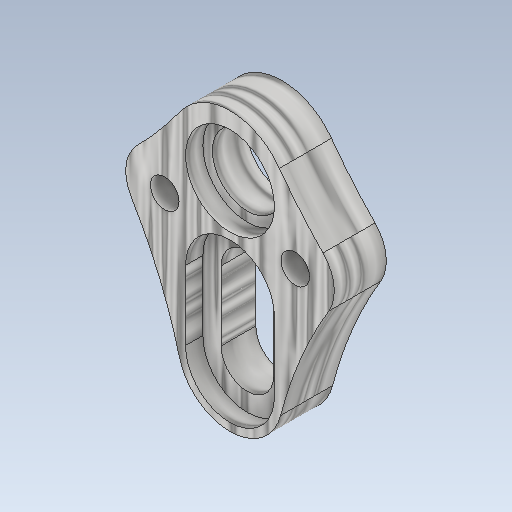
# Autodesk Inventor part: 横回転スライダー
Saved by Autodesk Inventor 2020 (Build 240168000, 168)
## iProperties
Created: 2019-09-03
Part Number: 横回転スライダー
Material: アルミニウム 7075
Document SubType Name: Modeling
Designer: tanjihayato
Density: 2.81 g/cm^3
Appearance: サテン - ブラシ仕上げ 重厚
Mass: 5.38037 g
Surface Area: 17.5615 cm^2
Volume: 1.91472 cm^3
Author: tanjihayato
Autodesk Inventor part; units mm, degrees
ref_plane "YZ Plane" through (0, 0, 0) normal (1, 0, 0) x (0, 1, 0)
ref_plane "XZ Plane" through (0, 0, 0) normal (0, 1, 0) x (-1, 0, 0)
ref_plane "XY Plane" through (0, 0, 0) normal (0, 0, 1) x (1, 0, 0)
sketch "スケッチ1" plane through (0, 0, 0) normal (0, 0, 1) x (1, 0, 0)
  circle A0 centre (0, 0) radius 4.025
  arc A1 (5.7008, 4.1051) -> (-5.7008, 4.1051) centre (0, 0) ccw
  line L0 (0, -11) -> (0, -19) construction
  line L1 (-3.025, -11) -> (-3.025, -19)
  line L2 (3.025, -19) -> (3.025, -11)
  arc A2 (3.025, -11) -> (-3.025, -11) centre (0, -11) ccw
  arc A3 (-3.025, -19) -> (3.025, -19) centre (0, -19) ccw
  arc A4 (-5.831, -20.5165) -> (5.831, -20.5165) centre (0, -19) ccw
  circle A5 centre (-7.525, -5) radius 1.65
  circle A6 centre (7.525, -5) radius 1.65
  line L3 (-7.525, -5) -> (7.525, -5) construction
  arc A7 (-10.7246, -1.8358) -> (-11.3806, -7.3203) centre (-7.525, -5) ccw
  arc A8 (-10.7246, -1.8358) -> (-5.7008, 4.1051) centre (-46.2759, 33.3226) ccw
  arc A9 (5.7008, 4.1051) -> (10.7246, -1.8358) centre (46.2759, 33.3226) ccw
  arc A10 (-5.831, -20.5165) -> (-11.3806, -7.3203) centre (-54.2212, -33.1019) ccw
  arc A11 (11.3806, -7.3203) -> (5.831, -20.5165) centre (54.2212, -33.1019) ccw
  arc A12 (11.3806, -7.3203) -> (10.7246, -1.8358) centre (7.525, -5) ccw
  point P0 (0, -15)
  dimension "d0" = 8.05
  dimension "d1" = 3
  dimension "d2" = 8
  dimension "d3" = 6.05
  dimension "d4" = 19
  dimension "d6" = 3.3
  dimension "d7" = 3.3
  dimension "d8" = 9
  dimension "d10" = 100
  dimension "d11" = 100
  dimension "d12" = 50
  dimension "d13" = 50
  dimension "d14" = 4.5
  dimension "d15" = 3
  dimension "d22" = 5
  constraints: 20 point on circle, 14 tangent, 13 centre point, 10 end point, 3 coincident, 1 horizontal, 1 midpoint, 1 parallel, 1 point on line, 1 vertical
  measures "d0" diameter of A0
  measures "d1" radial gap between concentric circles of A0 A1
  measures "d2" distance of L0.start L0.end
  measures "d3" diameter of A3
  measures "d4" distance of L0.end point (0, 0)
  measures "d6" diameter of A5
  measures "d7" diameter of A6
  measures "d8" diameter of A7
  measures "d10" diameter of A9
  measures "d11" diameter of A8
  measures "d12" radius of A11
  measures "d13" radius of A10
  measures "d14" radius of A12
  measures "d15" radial gap between concentric circles of A4 A3
  measures "d22" distance from line of L3 point (0, 0)
extrude "押し出し1" add sketch "スケッチ1" along normal blind 6
sketch "スケッチ2" plane through (0, 0, 6) normal (0, 0, 1) x (1, 0, 0)
  arc A0 (3.025, -11) -> (-3.025, -11) centre (0, -11) ccw projected
  line L0 (3.025, -11) -> (3.025, -19) projected
  arc A1 (-3.025, -19) -> (3.025, -19) centre (0, -19) ccw projected
  line L1 (-3.025, -19) -> (-3.025, -11) projected
  circle A2 centre (0, 0) radius 4.025 projected
  circle A3 centre (7.525, -5) radius 1.65 projected
  circle A4 centre (-7.525, -5) radius 1.65 projected
  arc A5 (-5.831, -20.5165) -> (5.831, -20.5165) centre (0, -19) ccw projected
  arc A6 (11.3806, -7.3203) -> (5.831, -20.5165) centre (54.2212, -33.1019) ccw projected
  arc A7 (11.3806, -7.3203) -> (10.7246, -1.8358) centre (7.525, -5) ccw projected
  arc A8 (5.7008, 4.1051) -> (10.7246, -1.8358) centre (46.2759, 33.3226) ccw projected
  arc A9 (5.7008, 4.1051) -> (-5.7008, 4.1051) centre (0, 0) ccw projected
  arc A10 (-10.7246, -1.8358) -> (-5.7008, 4.1051) centre (-46.2759, 33.3226) ccw projected
  arc A11 (-10.7246, -1.8358) -> (-11.3806, -7.3203) centre (-7.525, -5) ccw projected
  arc A12 (-5.831, -20.5165) -> (-11.3806, -7.3203) centre (-54.2212, -33.1019) ccw projected
  circle A13 centre (0, 0) radius 5.125
  arc A14 (5.125, -11) -> (-5.125, -11) centre (0, -11) ccw
  line L2 (5.125, -11) -> (5.125, -19)
  arc A15 (-5.125, -19) -> (5.125, -19) centre (0, -19) ccw
  line L3 (-5.125, -19) -> (-5.125, -11)
  dimension "d18" = 1.1
  dimension "d23" = 5.125
  constraints: 4 end point, 4 point on circle, 3 centre point, 3 other
  measures "d18" radial gap between concentric circles of A2 A13
  measures "d23" radius of A14
extrude "押し出し2" cut sketch "スケッチ2" against normal blind 2 contours A13 | L2 A15 L3 A14
